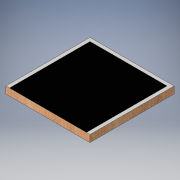
# Autodesk Inventor part: topStair
Saved by Autodesk Inventor 2016 (Build 200138000, 138)
## iProperties
Created: 2016-12-21
Part Number: topStair
Material: Wood (Birch)
Document SubType Name: Modeling
Designer: Naga
Density: 0.55 g/cm^3
Appearance: Birch - Natural Polished
Author: Naga
Autodesk Inventor part; units mm, degrees
ref_plane "YZ Plane" through (0, 0, 0) normal (1, 0, 0) x (0, 1, 0)
ref_plane "XZ Plane" through (0, 0, 0) normal (0, 1, 0) x (-1, 0, 0)
ref_plane "XY Plane" through (0, 0, 0) normal (0, 0, 1) x (1, 0, 0)
sketch "Sketch1" plane through (0, 0, 0) normal (0, 1, 0) x (-1, 0, 0)
  line L0 (0, 0) -> (304.8, 0)
  line L1 (304.8, 0) -> (304.8, -304.8)
  line L2 (304.8, -304.8) -> (0, -304.8)
  line L3 (0, -304.8) -> (0, 0)
  line L4 (12.7, -12.7) -> (292.1, -12.7)
  line L5 (292.1, -12.7) -> (292.1, -292.1)
  line L6 (292.1, -292.1) -> (12.7, -292.1)
  line L7 (12.7, -292.1) -> (12.7, -12.7)
  line L8 (12.7, -12.7) -> (292.1, -292.1) construction
  line L9 (292.1, -12.7) -> (12.7, -292.1) construction
  line L10 (12.7, -12.7) -> (0, -12.7)
  line L11 (12.7, -292.1) -> (0, -292.1)
  point P0 (152.4, -152.4)
  dimension "d0" = 304.8
  dimension "d1" = 304.8
  dimension "d2" = 279.4
  dimension "d3" = 279.4
  constraints: 24 end point, 4 parallel, 3 perpendicular, 3 point on line, 2 horizontal, 2 midpoint
  measures "d0" distance of L1.end L2.end
  measures "d1" distance of L0.end L1.end
  measures "d2" distance of L5.end L6.end
  measures "d3" distance of L4.end L5.end
extrude "Extrusion1" add sketch "Sketch1" along normal blind 25.4
sketch "Sketch2" plane through (0, 25.4, 0) normal (0, 1, 0) x (1, 0, 0)
  line L0 (-304.8, 0) -> (0, 0) projected
  line L1 (-152.4, 0) -> (-152.4, 304.8)
  line L2 (0, 0) -> (0, 304.8) projected
  line L3 (0, 152.4) -> (-304.8, 152.4)
  line L4 (-292.1, 12.7) -> (-12.7, 12.7)
  line L5 (-12.7, 12.7) -> (-12.7, 292.1)
  line L6 (-12.7, 292.1) -> (-292.1, 292.1)
  line L7 (-292.1, 292.1) -> (-292.1, 12.7)
  line L8 (-292.1, 12.7) -> (-12.7, 292.1) construction
  line L9 (-12.7, 12.7) -> (-292.1, 292.1) construction
  line L10 (-292.1, 12.7) -> (-292.1, 0)
  line L11 (-12.7, 12.7) -> (-12.7, 0)
  point P0 (-152.4, 152.4)
  dimension "d6" = 304.8
  dimension "d7" = 279.4
  dimension "d8" = 279.4
  constraints: 20 end point, 5 midpoint, 3 parallel, 2 horizontal, 2 perpendicular, 2 point on line, 1 vertical
  measures "d6" distance of L1.start L1.end
  measures "d7" distance of L6.end L5.end
  measures "d8" distance of L5.end L4.end
extrude "Extrusion2" cut sketch "Sketch2" against normal blind 0.0025 contours L10 L4 L1 L0 | L1 L4 L11 L0 | L7 L3 L1 L4 | L1 L3 L5 L4 | L7 L6 L1 L3 | L1 L6 L5 L3
body "Solid1"
